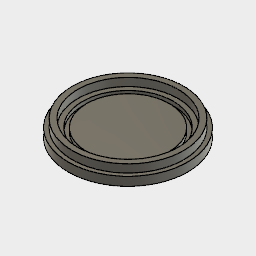
密封杯盖1 (Autodesk Fusion 360 design; units mm, degrees)
Autodesk Fusion 360 part; units mm, degrees
sketch "草图1" plane through (0, 0, 0) normal (0, 1, 0) x (1, 0, 0)
  circle A0 centre (0, 0) radius 35
  circle A1 centre (0, 0) radius 31
  dimension "d1" = 70
  dimension "d2" = 62
  measures "d1" diameter of A0
  measures "d2" diameter of A1
sketch "草图2" plane through (0, 5, 0) normal (0, 1, 0) x (-1, 0, 0)
  circle A0 centre (0, 0) radius 31
  circle A1 centre (0, 0) radius 35
  circle A2 centre (0, 0) radius 28.5
  circle A3 centre (0, 0) radius 26
  dimension "d5" = 57
  dimension "d6" = 52
  measures "d5" diameter of A2
  measures "d6" diameter of A3
sketch "草图3" plane through (0, 0, 0) normal (0, 1, 0) x (1, 0, 0)
sketch "草图4" plane through (0, 0, 0) normal (0, 1, 0) x (1, 0, 0)
  circle A0 centre (0, 0) radius 75
  dimension "d10" = 150
  measures "d10" diameter of A0
extrude "拉伸3" add sketch "草图4" along normal blind 11
sketch "草图5" plane through (0, 11, 0) normal (0, 1, 0) x (-1, 0, 0)
  circle A0 centre (0, 0) radius 75
  circle A1 centre (0, 0) radius 70
  circle A2 centre (0, 0) radius 63
  circle A3 centre (0, 0) radius 57
  circle A4 centre (0, 0) radius 52
  dimension "d13" = 140
  dimension "d15" = 126
  dimension "d16" = 114
  dimension "d17" = 104
  measures "d13" diameter of A1
  measures "d15" diameter of A2
  measures "d16" diameter of A3
  measures "d17" diameter of A4
extrude "拉伸4" add sketch "草图5" along normal blind 10 contours A1 | A3
extrude "拉伸6" cut 1 faces at (-54.9275, 21, -5.4152) along direction (0, -1, 0) blind 5
extrude "拉伸7" add 1 faces at (-54.9275, 16, -5.4152) along direction (0, -1, 0) blind 5
extrude "拉伸9" cut 1 faces at (-54.9275, 16, -5.4152) along direction (0, -1, 0) blind 10
extrude "拉伸8" [suppressed]
extrude "拉伸5" [suppressed]
